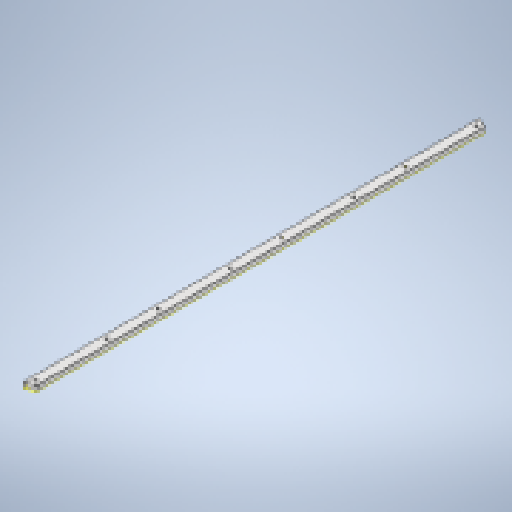
# Autodesk Inventor part: Long tube 1
Saved by Autodesk Inventor 2026.2 (Build 302298000, 298)
## iProperties
Created: 2026-05-21
Part Number: Long tube 1
Material: Generic
Document SubType Name: Modeling
Designer: admin
Density: 1 g/cm^3
Appearance: Default
Author: admin
Autodesk Inventor part; units mm, degrees
ref_plane "YZ Plane" through (0, 0, 0) normal (1, 0, 0) x (0, 1, 0)
ref_plane "XZ Plane" through (0, 0, 0) normal (0, 1, 0) x (-1, 0, 0)
ref_plane "XY Plane" through (0, 0, 0) normal (0, 0, 1) x (1, 0, 0)
sketch "Sketch1" plane through (0, 0, 0) normal (0, 0, 1) x (1, 0, 0)
  line L0 (-20, 10) -> (20, 10)
  line L1 (20, 10) -> (20, -10)
  line L2 (20, -10) -> (-20, -10)
  line L3 (-20, -10) -> (-20, 10)
  line L4 (-20, 10) -> (20, -10) construction
  line L5 (20, 10) -> (-20, -10) construction
  line L6 (18, 8) -> (-18, 8)
  line L7 (-18, 8) -> (-18, -8)
  line L8 (-18, -8) -> (18, -8)
  line L9 (18, -8) -> (18, 8)
  point P0 (0, 0)
  dimension "d0" = 40
  dimension "d1" = 20
  dimension "d2" = 2
  constraints: 20 end point, 4 parallel, 2 midpoint, 2 perpendicular, 1 horizontal, 3 other
  measures "d0" distance of L1.end L2.end
  measures "d1" distance of L0.end L1.end
  measures "d2" distance between parallel lines of L0 L6
extrude "Extrusion1" add sketch "Sketch1" along normal mid plane 1900
sketch "Sketch2" plane through (0, 0, 0) normal (0, 1, 0) x (-1, 0, 0)
  line L0 (20, -950) -> (20, 950) projected
  line L1 (-20, 950) -> (20, 950)
  line L2 (-20, -950) -> (-20, 950) projected
  line L3 (20, -950) -> (-20, -950) projected
  line L4 (-20, -950) -> (-50.7107, -950)
  line L5 (-50.7107, -950) -> (-50.7107, 950)
  line L6 (-50.7107, 950) -> (-20, 950)
  line L7 (20, -879.2893) -> (-50.7107, -950)
  line L8 (20, -879.2893) -> (-20, -862.7208)
  line L9 (-20, -950) -> (-20, 950) projected
  point P0 (0, 0)
  point P1 (-20, -919.2893)
  dimension "d5" = 45
  dimension "d6" = 100
  dimension "d19" = 67.5
  constraints: 12 end point, 2 perpendicular, 2 point on line, 1 horizontal
  measures "d5" angle of L4 L7
  measures "d6" distance of L7.start L4.end
  measures "d19" angle of L8 L7
extrude "Extrusion2" cut sketch "Sketch2" along normal through all both and the other way through all contours L3 L2 L7 L0 | L7 L2 L8
mirror "Mirror1" about plane through (0, 0, 0) normal (0, 0, 1) of "Extrusion2"
sketch "Sketch3" plane through (0, 0, 0) normal (0, 1, 0) x (-1, 0, 0)
  line L0 (0, 0) -> (0, -871.0051) construction
  line L1 (-20, -862.7208) -> (-20, 862.7208) construction
  line L2 (-20, -475) -> (20, -475) construction
  line L3 (20, 879.2893) -> (20, -879.2893) construction
  circle A0 centre (0, -100) radius 5.5
  circle A1 centre (0, -375) radius 5.5
  circle A2 centre (0, -575) radius 5.5
  circle A3 centre (0, -850) radius 5.5
  line L4 (20, 879.2893) -> (20, -879.2893) construction
  line L5 (-20, -862.7208) -> (20, -879.2893) construction
  dimension "d9" = 475
  dimension "d10" = 11
  dimension "d11" = 275
  dimension "d12" = 275
  dimension "d13" = 100
  dimension "d14" = 100
  dimension "d15" = 100
  constraints: 8 end point, 6 point on line, 4 centre point, 3 equal radius, 1 horizontal, 1 midpoint, 1 vertical
  measures "d9" distance from line of L0.start L2
  measures "d10" diameter of A0
  measures "d11" distance of A2.centre A3.centre
  measures "d12" distance of A1.centre A0.centre
  measures "d13" distance from line of L2 A2.centre
  measures "d14" distance of L0.start A0.centre
  measures "d15" distance from line of L2 A1.centre
extrude "Extrusion3" cut sketch "Sketch3" along normal through all
sketch "Sketch5" plane through (-20, -10, -879.2893) normal (0, -1, 0) x (1, 0, 0)
  line L0 (40, 1742.0101) -> (0, 1758.5786) construction
  line L1 (0, 1758.5786) -> (0, 0) construction
  line L2 (0, 0) -> (40, 16.5685) construction
  line L3 (40, 16.5685) -> (40, 1742.0101) construction
  circle A0 centre (20, 49.2893) radius 5.5
  point P0 (20, 879.2893)
  point P1 (20, 8.2843)
  dimension "d20" = 830
  dimension "d21" = 11
  constraints: 1 centre point, 1 midpoint, 1 vertical alignment
  measures "d20" distance of A0.centre point (20, 879.289)
  measures "d21" diameter of A0
extrude "Extrusion4" cut sketch "Sketch5" against normal up to surface (2 mm away)
mirror "Mirror2" about plane through (0, 0, 0) normal (0, 0, 1) of "Extrusion3", "Extrusion4"
fillet "Fillet1" radius 2 4 edges at (-20, 10, 0) (-20, -10, 0) (20, -10, 0) (20, 10, 0)
equation "\"d19\" = 1.5 * d5"
equation "\"d11\" = d12"
equation "\"d13\" = d15"
equation "\"d14\" = d15"
body "Solid1"
